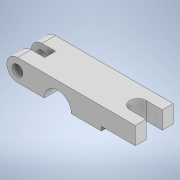
# Autodesk Inventor part: Plyta dociskowa
Saved by Autodesk Inventor 2021 (Build 250183000, 183)
## iProperties
Created: 2020-04-12
Part Number: Plyta dociskowa
Material: Ogólny
Document SubType Name: Modeling
Designer: dyrag
Density: 1 g/cm^3
Appearance: Domyślna
Author: dyrag
Autodesk Inventor part; units mm, degrees
ref_plane "YZ Plane" through (0, 0, 0) normal (1, 0, 0) x (0, 1, 0)
ref_plane "XZ Plane" through (0, 0, 0) normal (0, 1, 0) x (-1, 0, 0)
ref_plane "XY Plane" through (0, 0, 0) normal (0, 0, 1) x (1, 0, 0)
sketch "Szkic1" plane through (0, 0, 0) normal (0, 0, 1) x (1, 0, 0)
  line L0 (-28.581, 16.053) -> (52, 16.053)
  circle A0 centre (-35, 7.6573) radius 4
  line L1 (52, 16.053) -> (52, 3.053)
  line L2 (52, 3.053) -> (27, 3.053)
  line L3 (27, 3.053) -> (27, -0.0459)
  line L4 (27, -0.0459) -> (4.7982, -0.0459)
  arc A1 (4.7982, -0.0459) -> (-15.2013, 0.053) centre (-5.2013, 0.053) ccw
  line L5 (-28.581, 0.053) -> (-15.2013, 0.053)
  line L6 (-28.581, 0.053) -> (-34.9011, 0.053)
  line L7 (-28.581, 16.053) -> (-34.9011, 16.053)
  arc A2 (-34.9011, 16.053) -> (-34.9011, 0.053) centre (-34.9011, 8.053) ccw
  point P0 (0, 0)
  dimension "d1" = 8
  dimension "d2" = 20
  dimension "d3" = 25
  dimension "d4" = 52
  dimension "d6" = 13
  dimension "d7" = 87
  dimension "d8" = 16
  constraints: 16 end point, 4 horizontal, 4 point on circle, 3 centre point, 3 perpendicular, 2 tangent, 1 vertical, 4 other
  measures "d1" diameter of A0
  measures "d2" diameter of A1
  measures "d3" horizontal distance of L3.end L1.end
  measures "d4" distance from line of point (0, 0) L1
  measures "d6" distance of L1.end L0.end
  measures "d7" horizontal distance of A0.centre L1.end
  measures "d8" distance of L6.end L7.end
extrude "Wyciągnięcie proste1" add sketch "Szkic1" along normal mid plane 28
sketch "Szkic2" plane through (-34.9011, 16.053, 14) normal (0, 1, 0) x (1, 0, 0)
  line L0 (0, 28) -> (86.9011, 28) construction
  line L1 (86.9011, 0) -> (0, 0) construction
  line L2 (86.9011, 28) -> (86.9011, 0) construction
  line L3 (0, 28) -> (-8, 28) construction
  line L4 (-8, 0) -> (0, 0) construction
  line L5 (-8, 28) -> (-8, 0) construction
  line L6 (-8, 28) -> (-8, 0) construction
  line L7 (-8, 28) -> (-8, 0) construction
  line L8 (-8, 28) -> (-8, 0) construction
  line L9 (-8, 28) -> (-8, 0) construction
  line L10 (-8, 28) -> (-8, 0) construction
  line L11 (-8, 28) -> (-8, 0) construction
  line L12 (-8, 28) -> (-8, 0) construction
  line L13 (-8, 28) -> (-8, 0) construction
  line L14 (-8, 28) -> (-8, 0) construction
  line L15 (-8, 28) -> (-8, 0) construction
  line L16 (-8, 28) -> (-8, 0) construction
  line L17 (-8, 28) -> (-8, 0) construction
  line L18 (-8, 28) -> (-8, 0) construction
  line L19 (0, 28) -> (0, 0) construction
  line L20 (86.9011, 20) -> (74.9011, 20)
  line L21 (86.9011, 8) -> (74.9011, 8)
  arc A0 (74.9011, 20) -> (74.9011, 8) centre (74.9011, 14) ccw
  line L22 (10, 10) -> (10, 18)
  line L23 (10, 18) -> (-8, 18)
  line L24 (3.9011, 0) -> (3.9011, 28) projected
  line L25 (10, 10) -> (-8, 10)
  line L26 (-8, 18) -> (-8, 10)
  line L27 (86.9011, 20) -> (86.9011, 8)
  point P0 (34.9011, 14)
  dimension "d12" = 12
  dimension "d13" = 40
  dimension "d15" = 8
  dimension "d16" = 18
  constraints: 14 end point, 3 perpendicular, 2 point on circle, 2 tangent, 2 vertical, 1 centre point, 1 horizontal, 13 other
  measures "d12" distance of L21.start L20.start
  measures "d13" distance of A0.centre point (34.901, 14)
  measures "d15" distance of L25.end L23.end
  measures "d16" distance of L23.end L22.end
extrude "Wyciągnięcie proste2" cut sketch "Szkic2" against normal through all
